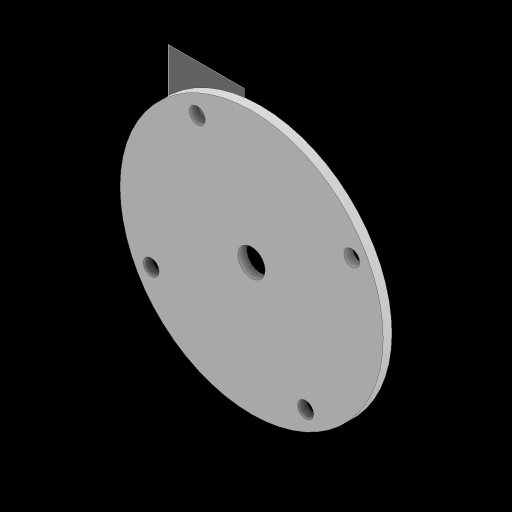
# Autodesk Inventor part: cover
Saved by Autodesk Inventor 2024.1 (Build 281209000, 209)
## iProperties
Created: 2025-05-13
Part Number: cover
Material: Generic
Document SubType Name: Modeling
Designer: Teddy
Density: 1 g/cm^3
Appearance: Default
Author: Teddy
Autodesk Inventor part; units mm, degrees
ref_plane "YZ Plane" through (0, 0, 0) normal (1, 0, 0) x (0, 1, 0)
ref_plane "XZ Plane" through (0, 0, 0) normal (0, 1, 0) x (-1, 0, 0)
ref_plane "Work Plane1" through (0, 0, 0) normal (0, 0, 1) x (1, 0, 0)
ref_plane "Work Plane2" through (-15.674, 29.0262, 3.81) normal (0, 0, 1) x (1, 0, 0)
sketch "Sketch2" plane through (-15.674, 29.0262, 3.81) normal (0, 0, 1) x (1, 0, 0)
  circle A0 centre (0, 0) radius 5.08 projected
  circle A1 centre (0, 0) radius 2.286 projected
  circle A2 centre (44.7003, -13.3522) radius 5.08 projected
  circle A3 centre (44.7003, -13.3522) radius 2.286 projected
  circle A4 centre (31.3481, -58.0524) radius 2.286 projected
  circle A5 centre (31.3481, -58.0524) radius 5.08 projected
  circle A6 centre (-13.3522, -44.7003) radius 2.286 projected
  circle A7 centre (-13.3522, -44.7003) radius 5.08 projected
  circle A8 centre (15.674, -29.0262) radius 38.0678
  circle A9 centre (15.674, -29.0262) radius 3.937
  dimension "d7" = 7.874
  constraints: 2 centre point, 2 coincident, 1 tangent
  measures "d7" diameter of A9
extrude "Extrusion2" add sketch "Sketch2" along normal blind 2.54 contours A0 | A7 | A5 | A2 | A8
body "Solid1"
